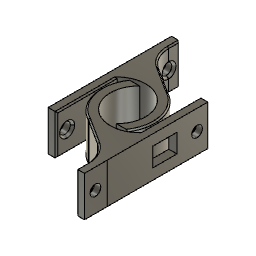
Gancicno osscuranti finestre v2 (Autodesk Fusion 360 design; units mm, degrees)
Autodesk Fusion 360 part; units mm, degrees
note: some values were not read from the file. Set by a fixed rule: which sketch regions a step uses.
sketch "Schizzo1" plane through (0, 0, 0) normal (1, 0, 0) x (0, 1, 0)
  line L0 (30.0466, 3.0565) -> (-0.0091, 2.9642)
  line L1 (-0.0091, 2.9642) -> (40, 3.0871)
  line L2 (0, 0) -> (40, 0)
  line L3 (40, 3.0871) -> (40, 0)
  line L4 (0, 0) -> (-0.0091, 2.9642)
  circle A0 centre (22.3372, 10.5) radius 10.6593 construction
  circle A1 centre (22.3372, 10.5) radius 14 construction
  line L5 (30, 18.2248) -> (29.9877, 22.2247) construction
  line L6 (9.8276, 16.7858) -> (1.0193, 2.9673) construction
  circle A2 centre (22.3372, 10.5) radius 10.6593
  circle A3 centre (22.3372, 10.5) radius 14
  line L7 (1.0193, 2.9673) -> (10.1744, 17.3297)
  line L8 (29.9877, 22.2247) -> (30, 18.2248)
  line L9 (29.9877, 22.2247) -> (30.001, 17.9085)
  dimension "d19" = 28
  constraint parallel L0 L1
  constraint coincident L2.start L4.start
  constraint horizontal L2
  constraint perpendicular L2 L3
  constraint perpendicular L1 L4
  constraint concentric A0 A1
  constraint coincident A1 L5.end
  constraint coincident A1 L6.start
  constraint coincident L1 L6.end
  constraint concentric A0 A2
  constraint concentric A2 A3
  constraint parallel L6 L7
  constraint parallel L5 L8
  constraint coincident A2 L9.end
  constraint parallel L8 L9
  measures "d19" diameter of A1
extrude "Estrusione5" add sketch "Schizzo1" along normal blind 15 contours L0 L1 L2 L4 A3 | L0 L1 A3 L7 | L0 L1 A2 A3 L8 L9 | L0 L1 L2 A2 A3 | L0 L1 L2 A2 | L0 L1 L2 A2 A3 | L1 L2 L3 A3 picked at (11.0025, 4.4227) makes body 1
extrude "Estrusione6" add 1 faces at (10, -0.003, 0.9881) along direction (0, -0.999995, -0.003073) blind 9 on bodies 1 bodies 1
extrude "Estrusione7" cut 1 faces at (5, 40, 2.0581) along direction (0, -1, 0) blind 2.5 on bodies 1 bodies 1
extrude "Estrusione8" cut 1 faces at (10, -9.003, 0.9604) along direction (0, 0.999995, 0.003073) blind 2.5 on bodies 1 bodies 1
extrude "Estrusione9" add 1 faces at (10, -6.503, 0.9681) along direction (0, -0.999995, -0.003073) blind 2 on bodies 1 bodies 1
fillet "Raccordo2" radius 10 2 edges at (7.5, 1.0193, 2.9673) (7.5, 9.8276, 16.7858) on bodies 1
sketch "Schizzo5" plane through (0, 0, 0) normal (0, 0, 1) x (1, 0, 0)
  line L0 (4, 26) -> (11, 26)
  line L1 (11, 26) -> (11, 13)
  line L2 (11, 13) -> (4, 13)
  line L3 (4, 13) -> (4, 26)
  line L4 (11, 17) -> (4, 17)
  line L5 (4, 17) -> (4, 26)
  line L6 (4, 26) -> (11, 26)
  line L7 (11, 26) -> (11, 17)
  constraint horizontal L0
  constraint vertical L1
  constraint horizontal L2
  constraint vertical L3
  constraint horizontal L4
  constraint vertical L5
  constraint horizontal L6
  constraint vertical L7
  constraint coincident L1 L4.start
extrude "Estrusione10" cut sketch "Schizzo5" along normal blind 5 contours L0 L1 L3 L4 L5 L6 L7 bodies 1
sketch "Schizzo6" plane through (0, 0, 0) normal (0, 0, 1) x (1, 0, 0)
  line L0 (15, 30) -> (15, 37)
  circle A0 centre (7.5, 33.5) radius 2
  circle A1 centre (7.5, -4.4245) radius 2
  dimension "d35" = 4
  dimension "d36" = 4
  constraint vertical L0
  measures "d35" diameter of A0
  measures "d36" diameter of A1
extrude "Estrusione11" cut sketch "Schizzo6" along normal blind 5 contours A1 bodies 1
extrude "Estrusione12" cut 1 faces at (8.0508, -4.6275, 0) along direction (0, 0, -1) blind 3 on bodies 1 bodies 1
extrude "Estrusione13" cut sketch "Schizzo6" along normal blind 6 contours A0 bodies 1
chamfer "Smusso3" distance 0.8 angle 45 3 edges at (7.5, -2.4245, 3.1632) (7.5, -6.4245, 2.9444) (7.5, 31.5, 3.061) measured on face at (7.4853, -0.9843, 3.5799) measured on face at (1.8972, -6.0778, 2.9455) measured on face at (1.3333, 26.0845, 3.0443) on bodies 1
chamfer "Smusso4" distance 0.5 angle 45 14 edges at (7.5, 37.5, 3.0794) (0, 26.1267, 3.0445) (15, 26.1267, 3.0445) (15, -6.4772, 2.9443) (15, 18.8535, 24.0596) (15, 9.793, 16.7455) (15, 6.7735, 11.9944) (15, 0.3463, 4.19) (0, -6.4772, 2.9443) (0, 0.3463, 4.19) (0, 6.7735, 11.9944) (0, 9.793, 16.7455) (0, 18.8535, 24.0596) (7.5, -8.5091, 2.938) measured on face at (1.3333, 26.0845, 3.0443) measured on face at (0, 5.2869, 3.1951) measured on face at (15, 5.2869, 3.1951) measured on face at (15, 5.2869, 3.1951) measured on face at (15, 5.2869, 3.1951) measured on face at (5, 9.9416, 17.009) measured on face at (15, 5.2869, 3.1951) measured on face at (7.5334, -0.736, 3.6762) measured on face at (0, 5.2869, 3.1951) measured on face at (7.5334, -0.736, 3.6762) measured on face at (0, 5.2869, 3.1951) measured on face at (5, 9.9416, 17.009) measured on face at (10, 16.4268, 23.1912) measured on face at (10, -8.503, 0.9619) on bodies 1
move_body "Sposta2" bodies 1 to x (0, 0, 1) y (0, 1, 0) z (-1, 0, 0) at (0, 0, 0)
copy_body "CopiaIncollaCorpi1" bodies 1 makes body 2
move_body "Sposta3" bodies 2 to x (-1, 0, 0) y (0, -1, 0) z (0, 0, 1) at (-28, 43.4849, 0)
combine "Combina1" operation add target body 1 tool bodies 2 makes body 3 at (-9.38, 14.2423, 10)
move_body "Sposta1" [rolled back]
sketch "Schizzo4" plane through (0, 0, 0) normal (1, 0, 0) x (0, 1, 0)
  circle A0 centre (22.5, 10.5) radius 14.3
  line L0 (30, 22) -> (29.9808, 22)
  line L1 (29.9808, 22.6872) -> (30, 22.6872)
  line L2 (29.9843, 22.2246) -> (29.9808, 22.6872)
  dimension "d32" = 28.6
  constraint horizontal L0
  constraint horizontal L1
  constraint coincident A0 L1.start
  measures "d32" diameter of A0
